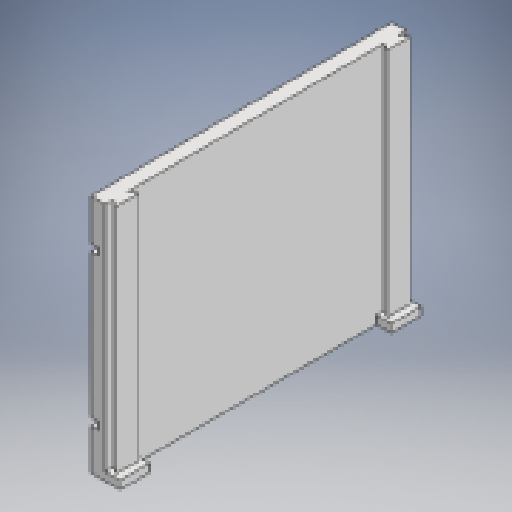
# Autodesk Inventor part: drawerside
Saved by Autodesk Inventor 2025.2 (Build 292293000, 293)
## iProperties
Created: 2025-02-24
Part Number: drawerside
Material: Generic
Document SubType Name: Modeling
Designer: email
Density: 1 g/cm^3
Appearance: Default
Author: email
Autodesk Inventor part; units mm, degrees
ref_plane "YZ Plane" through (0, 0, 0) normal (1, 0, 0) x (0, 1, 0)
ref_plane "XZ Plane" through (0, 0, 0) normal (0, 1, 0) x (-1, 0, 0)
ref_plane "XY Plane" through (0, 0, 0) normal (0, 0, 1) x (1, 0, 0)
sketch "Sketch1" plane through (0, 0, 0) normal (0, 1, 0) x (-1, 0, 0)
  line L0 (0, 0) -> (0, -100)
  line L1 (0, -100) -> (-5, -100)
  line L2 (-5, -100) -> (-5, -97.5)
  line L3 (-5, -92.5) -> (-5, -7.5)
  line L4 (-5, -7.5) -> (-7.5, -9)
  line L5 (-7.5, -9) -> (-7.5, -1)
  line L6 (-7.5, -1) -> (-5, -2.5)
  line L7 (-5, -2.5) -> (-5, 0)
  line L8 (-5, 0) -> (0, 0)
  line L9 (-5, -7.5) -> (-5, -2.5) construction
  line L10 (-5, -92.5) -> (-5, -97.5) construction
  line L11 (0, -50) -> (-5, -50) construction
  line L12 (-5, -92.5) -> (-7.5, -91)
  line L13 (-7.5, -91) -> (-7.5, -99)
  line L14 (-7.5, -99) -> (-5, -97.5)
  line L15 (0, 0) -> (-10, 0)
  line L16 (-10, 0) -> (-10, -10)
  line L17 (-10, -10) -> (0, -10)
  line L18 (0, -10) -> (0, 0)
  line L19 (0, -100) -> (-10, -100)
  line L20 (-10, -100) -> (-10, -90)
  line L21 (-10, -90) -> (0, -90)
  line L22 (0, -90) -> (0, -100)
  point P0 (-7.5, -5)
  point P1 (-5, -5)
  point P2 (-5, -95)
  point P3 (0, -90)
  point P4 (-5, 0)
  point P5 (0, -10)
  point P6 (-5, -90)
  dimension "d0" = 100
  dimension "d1" = 5
  dimension "d2" = 8
  dimension "d3" = 5
  dimension "d4" = 5
  dimension "d5" = 2.5
  dimension "d6" = 5
  dimension "d9" = 5
  dimension "d10" = 10
  dimension "d11" = 10
  dimension "d12" = 10
  dimension "d13" = 10
  constraints: 46 end point, 5 midpoint, 5 parallel, 5 perpendicular, 4 vertical, 2 horizontal, 2 point on line, 2 symmetric about line, 1 collinear, 1 horizontal alignment
  measures "d0" distance between parallel lines of L1 L8
  measures "d1" distance between parallel lines of L0 L3
  measures "d2" distance of L4.end L5.end
  measures "d3" distance of L6.end L3.end
  measures "d4" distance from line of L8 point (-7.5, -5)
  measures "d5" distance between parallel lines of L7 L5
  measures "d6" distance of L3.start L2.end
  measures "d9" distance from line of L1 point (-5, -95)
  measures "d10" distance of L0.start L15.end
  measures "d11" distance of L15.end L16.end
  measures "d12" distance of L20.end L21.end
  measures "d13" distance of L19.end L20.end
extrude "Extrusion1" add sketch "Sketch1" along normal blind 3 contours L0 L17 L3 L4 L5 L6 L7 L8 | L7 L6 L5 L4 L3 L17 L16 L15 | L0 L1 L2 L14 L13 L12 L3 L21 | L3 L12 L13 L14 L2 L19 L20 L21
extrude "Extrusion2" add sketch "Sketch1" along normal blind 80 contours L0 L17 L3 L4 L5 L6 L7 L8 | L0 L21 L3 L17 | L0 L1 L2 L14 L13 L12 L3 L21
sketch "Sketch2" plane through (0, 0, 0) normal (0, 0, 1) x (1, 0, 0)
  line L0 (0, 0) -> (0, 80) projected
  line L1 (0, 13.75) -> (2.5, 13.75)
  line L2 (2.5, 13.75) -> (2.5, 16.25)
  line L3 (2.5, 16.25) -> (0, 16.25)
  line L4 (0, 16.25) -> (0, 13.75)
  line L5 (0, 66.25) -> (2.5, 66.25)
  line L6 (2.5, 66.25) -> (2.5, 63.75)
  line L7 (2.5, 63.75) -> (0, 63.75)
  line L8 (0, 63.75) -> (0, 66.25)
  line L9 (0, 80) -> (5, 80) projected
  line L10 (0, 0) -> (10, 0) projected
  point P0 (2.5, 65)
  point P1 (2.5, 15)
  point P2 (0, 16.25)
  dimension "d18" = 15
  dimension "d19" = 2.5
  dimension "d20" = 2.5
  dimension "d21" = 15
  dimension "d22" = 2.5
  constraints: 16 end point, 4 parallel, 3 point on line, 2 horizontal, 2 midpoint, 2 perpendicular
  measures "d18" distance from line of L9 point (2.5, 65)
  measures "d19" distance of L5.end L6.end
  measures "d20" distance between parallel lines of L0 L6
  measures "d21" distance from line of L10 point (2.5, 15)
  measures "d22" distance between parallel lines of L1 L3
extrude "Extrusion3" cut sketch "Sketch2" against normal up to surface (100 mm away)
sketch "Sketch3" plane through (0, 3, 0) normal (0, 1, 0) x (1, 0, 0)
  line L0 (5, 92.5) -> (5, 90) projected
  line L1 (5, 90) -> (10, 90) projected
  line L2 (10, 90) -> (10, 100) projected
  line L3 (10, 100) -> (5, 100) projected
  line L4 (5, 100) -> (5, 97.5) projected
  line L5 (5, 97.5) -> (7.5, 99) projected
  line L6 (7.5, 99) -> (7.5, 91) projected
  line L7 (7.5, 91) -> (5, 92.5) projected
  line L8 (5, 10) -> (5, 7.5) projected
  line L9 (5, 7.5) -> (7.5, 9) projected
  line L10 (7.5, 9) -> (7.5, 1) projected
  line L11 (7.5, 1) -> (5, 2.5) projected
  line L12 (5, 2.5) -> (5, 0) projected
  line L13 (5, 0) -> (10, 0) projected
  line L14 (10, 0) -> (10, 10) projected
  line L15 (10, 10) -> (5, 10) projected
  point P0 (0, 0)
extrude "Extrusion4" cut sketch "Sketch3" against normal blind 0.1
sketch "Sketch4" plane through (0, 80, 0) normal (0, 1, 0) x (1, 0, 0)
  line L0 (7.5, 99) -> (5, 97.5) projected
  line L1 (7.5, 91) -> (7.5, 99) projected
  line L2 (5, 92.5) -> (7.5, 91) projected
  line L3 (7.5, 9) -> (5, 7.5) projected
  line L4 (7.5, 1) -> (7.5, 9) projected
  line L5 (5, 2.5) -> (7.5, 1) projected
  line L6 (5, 7.3834) -> (7.4, 8.8234)
  line L7 (7.4, 8.8234) -> (7.4, 1.1766)
  line L8 (7.4, 1.1766) -> (5, 2.6166)
  line L9 (5, 92.6166) -> (7.4, 91.1766)
  line L10 (7.4, 91.1766) -> (7.4, 98.8234)
  line L11 (7.4, 98.8234) -> (5, 97.3834)
  line L12 (5, 7.5) -> (5, 92.5) projected
  line L13 (5, 97.5) -> (5, 92.5)
  line L14 (5, 7.5) -> (5, 2.5)
  point P0 (0, 0)
  dimension "d27" = 0.1
  dimension "d28" = 0.1
  dimension "d29" = 0.1
  dimension "d30" = 0.1
  dimension "d33" = 0.1
  dimension "d34" = 0.1
  constraints: 16 end point, 4 point on line, 1 collinear, 1 vertical
  measures "d27" distance between parallel lines of L4 L7
  measures "d28" distance between parallel lines of L2 L9
  measures "d29" distance between parallel lines of L1 L10
  measures "d30" distance between parallel lines of L0 L11
  measures "d33" distance between parallel lines of L3 L6
  measures "d34" distance between parallel lines of L5 L8
extrude "Extrusion5" cut sketch "Sketch4" against normal up to surface (77.1 mm away) contours L1 L2 L13 L9 L10 L11 L0 | L4 L5 L14 L8 L7 L6 L3
sketch "Sketch5" plane through (10, 0, -90) normal (1, 0, 0) x (0, 0, -1)
  line L0 (-80, 2.9) -> (-90, 2.9) projected
  line L1 (-90, 0) -> (-90, 2.9) projected
  line L2 (-90, 0) -> (-80, 0) projected
  line L3 (-80, 0) -> (-80, 2.9) projected
  line L4 (10, 2.9) -> (0, 2.9) projected
  line L5 (0, 0) -> (0, 2.9) projected
  line L6 (0, 0) -> (10, 0) projected
  line L7 (10, 0) -> (10, 2.9) projected
extrude "Extrusion6" cut sketch "Sketch5" against normal blind 0.1
sketch "Sketch6" plane through (9.9, 0, -90) normal (1, 0, 0) x (0, 0, -1)
  line L0 (10, 0) -> (-90, 0) projected
  line L1 (-81.1766, 2.9) -> (-88.8234, 2.9) projected
  line L2 (0.1, 0) -> (-80.1, 0)
  line L3 (-80.1, 0) -> (-80.1, 2.9)
  line L4 (-80.1, 2.9) -> (0.1, 2.9)
  line L5 (0.1, 2.9) -> (0.1, 0)
  line L6 (-80, 2.9) -> (-80, 0) construction
  line L7 (0, 0) -> (0, 2.9) construction
  dimension "tol" = 0.1
  dimension "d38" = 0.1
  constraints: 8 end point, 2 parallel, 2 point on line, 1 horizontal, 1 perpendicular
  measures "tol" distance between parallel lines of L3 L6
  measures "d38" distance between parallel lines of L7 L5
extrude "Extrusion7" cut sketch "Sketch6" against normal up to surface (4.9 mm away)
sketch "Sketch7" plane through (0, 80, 0) normal (0, 1, 0) x (1, 0, 0)
  line L0 (5, 97.3834) -> (5, 100) projected
  line L1 (5, 100) -> (0, 100) projected
  line L2 (0, 100) -> (0, 0) projected
  line L3 (0, 0) -> (5, 0) projected
  line L4 (5, 0) -> (5, 2.6166) projected
  line L5 (5, 2.6166) -> (7.4, 1.1766) projected
  line L6 (7.4, 1.1766) -> (7.4, 8.8234) projected
  line L7 (7.4, 8.8234) -> (5, 7.3834) projected
  line L8 (5, 7.3834) -> (5, 92.6166) projected
  line L9 (5, 92.6166) -> (7.4, 91.1766) projected
  line L10 (7.4, 91.1766) -> (7.4, 98.8234) projected
  line L11 (7.4, 98.8234) -> (5, 97.3834) projected
extrude "Extrusion8" cut sketch "Sketch7" against normal blind 0.2
sketch "Sketch8" plane through (0, 0, 0) normal (0, -1, 0) x (1, 0, 0)
  line L0 (5, -9.9) -> (9.9, -9.9) projected
  line L1 (9.9, -9.9) -> (9.9, 0) projected
  line L2 (0, 0) -> (9.9, 0) projected
  line L3 (0, -100) -> (0, 0) projected
  line L4 (9.9, -100) -> (0, -100) projected
  line L5 (9.9, -100) -> (9.9, -90.1) projected
  line L6 (9.9, -90.1) -> (5, -90.1) projected
  line L7 (5, -90.1) -> (5, -9.9) projected
extrude "Extrusion9" cut sketch "Sketch8" against normal blind 0.2
sketch "Sketch9" plane through (0, 16.25, 0) normal (-1, 0, 0) x (0, 0, 1)
  line L0 (-100, 0) -> (0, 0) projected
  line L1 (0, 0) -> (0, 47.5) projected
  line L2 (0, 47.5) -> (-100, 47.5) projected
  line L3 (-100, 0) -> (-100, 47.5) projected
  line L4 (0, 63.55) -> (-100, 63.55) projected
  line L5 (-100, 50) -> (-100, 63.55) projected
  line L6 (-100, 50) -> (0, 50) projected
  line L7 (0, 50) -> (0, 63.55) projected
  line L8 (-100, -16.05) -> (0, -16.05) projected
  line L9 (0, -16.05) -> (0, -2.5) projected
  line L10 (0, -2.5) -> (-100, -2.5) projected
  line L11 (-100, -16.05) -> (-100, -2.5) projected
  point P0 (0, -16.25)
extrude "Extrusion10" cut sketch "Sketch9" against normal blind 0.2
equation "\"d25\" = tol"
equation "\"d27\" = tol"
equation "\"d28\" = tol"
equation "\"d29\" = tol"
equation "\"d30\" = tol"
equation "\"d33\" = tol"
equation "\"d34\" = tol"
equation "\"d35\" = tol"
equation "\"d38\" = tol"
equation "\"d41\" = 2 * tol"
equation "\"d43\" = 2 * tol"
equation "\"d45\" = 2 * tol"
body "Solid1"
